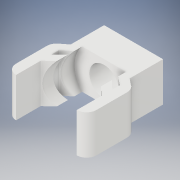
# Autodesk Inventor part: Arm8
Saved by Autodesk Inventor 2017 SP1 (Build 210196100, 196)
## iProperties
Created: 2018-02-11
Part Number: Arm8
Material: ABS Plastic
Document SubType Name: Modeling
Designer: Zach
Density: 1.06 g/cm^3
Appearance: CR White
Author: Zach
Autodesk Inventor part; units mm, degrees
ref_plane "YZ Plane" through (0, 0, 0) normal (1, 0, 0) x (0, 1, 0)
ref_plane "XZ Plane" through (0, 0, 0) normal (0, 1, 0) x (-1, 0, 0)
ref_plane "XY Plane" through (0, 0, 0) normal (0, 0, 1) x (1, 0, 0)
sketch "Sketch1" plane through (0, 0, 0) normal (0, 0, 1) x (1, 0, 0)
  circle A0 centre (0, 0) radius 1.5
  line L0 (-3, 2) -> (3, 2)
  line L1 (3, 2) -> (3, -2)
  line L2 (3, -2) -> (-3, -2)
  line L3 (-3, -2) -> (-3, 2)
  point P0 (-3, 0)
  point P1 (0, 2)
  dimension "d0" = 3
  dimension "d1" = 6
  dimension "d2" = 4
  constraints: 8 end point, 2 midpoint, 2 parallel, 1 centre point, 1 coincident, 1 horizontal, 1 horizontal alignment, 1 perpendicular, 1 vertical alignment
  measures "d0" diameter of A0
  measures "d1" distance of L1.end L2.end
  measures "d2" distance of L0.end L1.end
extrude "Extrusion1" add sketch "Sketch1" along normal blind 2
sketch "Sketch2" plane through (-3, 2, 0) normal (0, 1, 0) x (1, 0, 0)
  line L0 (6, -2) -> (0, -2) projected
  line L1 (1.75, -2) -> (4.25, -2)
  line L2 (4.25, -2) -> (4.25, -5)
  line L3 (4.25, -5) -> (1.75, -5)
  line L4 (1.75, -5) -> (1.75, -2)
  line L5 (-0.0919, -3.875) -> (-1.0919, -3.875)
  line L6 (-1.0919, -3.875) -> (-1.0919, -8.875)
  line L7 (-1.0919, -8.875) -> (-0.0919, -8.875)
  line L8 (-0.0919, -8.875) -> (-0.0919, -3.875)
  line L9 (-0.5919, -3.875) -> (1.75, -2) construction
  line L10 (1.75, -2) -> (2.25, -2.6245) construction
  line L11 (2.25, -2.6245) -> (-0.0919, -4.4995) construction
  line L12 (-0.0919, -4.4995) -> (-0.5919, -3.875) construction
  line L13 (-0.0919, -6.375) -> (2.3038, -4.0774) construction
  line L14 (2.3038, -4.0774) -> (1.75, -3.5) construction
  line L15 (1.75, -3.5) -> (-0.6456, -5.7976) construction
  line L16 (-0.6456, -5.7976) -> (-0.0919, -6.375) construction
  line L17 (6.0919, -8.875) -> (7.0919, -8.875)
  line L18 (7.0919, -8.875) -> (7.0919, -3.875)
  line L19 (7.0919, -3.875) -> (6.0919, -3.875)
  line L20 (6.0919, -3.875) -> (6.0919, -8.875)
  line L21 (4.25, -2) -> (6.5919, -3.875) construction
  line L22 (6.5919, -3.875) -> (6.0919, -4.4995) construction
  line L23 (6.0919, -4.4995) -> (3.75, -2.6245) construction
  line L24 (3.75, -2.6245) -> (4.25, -2) construction
  line L25 (6.0919, -6.375) -> (3.6962, -4.0774) construction
  line L26 (3.6962, -4.0774) -> (4.25, -3.5) construction
  line L27 (4.25, -3.5) -> (6.6456, -5.7976) construction
  line L28 (6.6456, -5.7976) -> (6.0919, -6.375) construction
  line L29 (-0.0919, -6.375) -> (1.75, -4.6085)
  line L30 (-0.0919, -6.375) -> (-0.0919, -5.2665)
  line L31 (-0.0919, -5.2665) -> (1.75, -3.5)
  line L32 (1.75, -3.5) -> (1.75, -4.6085)
  line L33 (-0.0919, -4.4995) -> (-0.0919, -3.875)
  line L34 (-0.0919, -3.875) -> (-0.5919, -3.875)
  line L35 (-0.5919, -3.875) -> (1.75, -2)
  line L36 (1.75, -2) -> (1.75, -3.0248)
  line L37 (1.75, -3.0248) -> (-0.0919, -4.4995)
  line L38 (6.0919, -6.375) -> (6.0919, -5.2665)
  line L39 (6.0919, -5.2665) -> (4.25, -3.5)
  line L40 (4.25, -3.5) -> (4.25, -4.6085)
  line L41 (4.25, -4.6085) -> (6.0919, -6.375)
  line L42 (4.25, -3.0248) -> (6.0919, -4.4995)
  line L43 (6.0919, -4.4995) -> (6.0919, -3.875)
  line L44 (6.0919, -3.875) -> (6.5919, -3.875)
  line L45 (6.5919, -3.875) -> (4.25, -2)
  line L46 (4.25, -2) -> (4.25, -3.0248)
  point P0 (3, 0)
  point P1 (3, -2)
  dimension "d5" = 2.5
  dimension "d6" = 3
  dimension "d7" = 1
  dimension "d8" = 5
  dimension "d11" = 0.8
  dimension "d13" = 3
  dimension "d15" = 0.8
  dimension "d18" = 1
  dimension "d19" = 5
  dimension "d20" = 0.8
  dimension "d21" = 3
  dimension "d22" = 0.8
  constraints: 92 end point, 17 parallel, 14 point on line, 10 perpendicular, 8 midpoint, 4 collinear, 3 horizontal, 1 horizontal alignment
  measures "d5" distance of L2.end L3.end
  measures "d6" distance of L1.end L2.end
  measures "d7" distance of L7.end L6.end
  measures "d8" distance of L6.end L5.end
  measures "d11" distance between parallel lines of L9 L11
  measures "d13" distance of L9.start L1.start
  measures "d15" distance between parallel lines of L15 L13
  measures "d18" distance of L19.end L18.end
  measures "d19" distance of L18.end L17.end
  measures "d20" distance of L23.end L1.end
  measures "d21" distance of L1.end L21.end
  measures "d22" distance of L26.end L25.end
extrude "Extrusion3" add sketch "Sketch2" against normal blind 4 contours L2 L3 L4 L0 | L45 L19 L20 L42 L2 | L4 L37 L8 L5 L35 | L19 L18 L17 L20 | L5 L8 L7 L6 | L39 L20 L41 L2 | L4 L29 L8 L31
fillet "Fillet1" radius 1 6 edges at (-4.0919, 0, 8.875) (4.0919, 0, 8.875) (4.0919, 0, 3.875) (-4.0919, 0, 3.875) (-1.25, 0, 5) (1.25, 0, 5)
sketch "Sketch5" plane through (-3, 2, 0) normal (0, 1, 0) x (1, 0, 0)
  line L0 (1.75, -2) -> (0, -2) projected
  line L1 (0, -2) -> (0, -3.4011)
  line L2 (1.75, -2) -> (-0.5919, -3.875) projected
  line L3 (1.75, -2) -> (0, -3.4011)
  line L4 (6, -2) -> (6, -3.4011)
  line L5 (4.25, -2) -> (1.75, -2) projected
  line L6 (6, -3.4011) -> (4.25, -2)
  line L7 (4.25, -2) -> (6, -2)
  line L8 (6.5919, -3.875) -> (4.25, -2) projected
  point P0 (3, 0)
  constraints: 10 end point, 2 collinear, 2 point on line, 2 vertical
extrude "Extrusion4" add sketch "Sketch5" against normal blind 4
sketch "Sketch6" plane through (0, 0, 0) normal (0, 0, -1) x (-1, 0, 0)
  circle A0 centre (0, 0) radius 1.5 projected
extrude "Extrusion5" cut sketch "Sketch6" against normal through all
sketch "Sketch7" plane through (-0.4564, 2, 5) normal (0, 0, 1) x (1, 0, 0)
  circle A0 centre (0.4564, -2) radius 3
  dimension "d31" = 6
  constraints: 1 centre point, 1 coincident
  measures "d31" diameter of A0
extrude "Extrusion6" cut sketch "Sketch7" along normal mid plane 4
body "Solid1"
